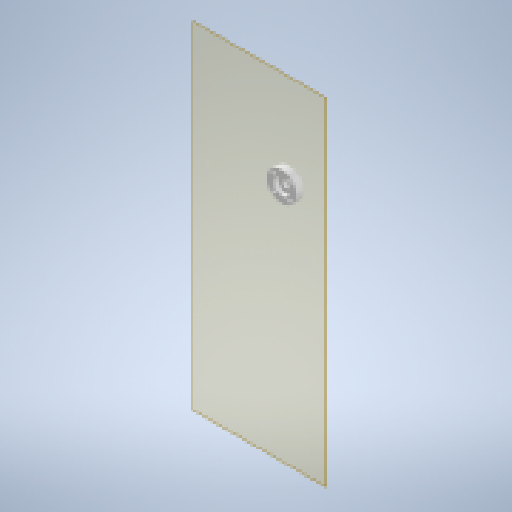
# Autodesk Inventor part: подшипник не выпадет
Saved by Autodesk Inventor 2024.2 (Build 282272000, 272)
## iProperties
Created: 2026-03-10
Part Number: подшипник не выпадет
Material: Типовые
Document SubType Name: Modeling
Designer: Service
Density: 1 g/cm^3
Appearance: По умолчанию
Author: Service
Autodesk Inventor part; units mm, degrees
ref_plane "YZ Plane" through (0, 0, 0) normal (1, 0, 0) x (0, 1, 0)
ref_plane "XZ Plane" through (0, 0, 0) normal (0, 1, 0) x (-1, 0, 0)
ref_plane "XY Plane" through (0, 0, 0) normal (0, 0, 1) x (1, 0, 0)
ref_plane "РабПлоскость1" through (0, 0, 0) normal (0, 0, 1) x (1, 0, 0)
sketch "Эскиз1" plane through (0, 0, 0) normal (0, 0, 1) x (1, 0, 0)
  circle A0 centre (30, 88.544) radius 1.5 projected
  circle A1 centre (30, 74.544) radius 1.5 projected
  circle A2 centre (16, 74.544) radius 1.5 projected
  circle A3 centre (16, 88.544) radius 1.5 projected
  circle A4 centre (23, 81.544) radius 7 projected
  circle A5 centre (23, 81.544) radius 12.5
  circle A6 centre (23, 81.544) radius 3
  point P0 (0, 0)
  dimension "d0" = 25
  dimension "d5" = 6
  constraints: 2 centre point, 2 coincident
  measures "d0" diameter of A5
  measures "d5" diameter of A6
extrude "Выдавливание1" add sketch "Эскиз1" along normal blind 6 contours A5
extrude "Выдавливание2" add sketch "Эскиз1" along normal blind 2 contours A4
